rotary bearing mount_v3 (Autodesk Fusion 360 design; units mm, degrees)
Autodesk Fusion 360 part; units mm, degrees
sketch "Sketch1" plane through (0, 0, 0) normal (0, 0, 1) x (1, 0, 0)
  line L0 (-45, 45) -> (45, 45) construction
  line L1 (45, 45) -> (45, -45) construction
  line L2 (45, -45) -> (-45, -45) construction
  line L3 (-45, -45) -> (-45, 45) construction
  line L4 (-45, 45) -> (45, -45) construction
  line L5 (45, 45) -> (-45, -45) construction
  circle A0 centre (-45, 45) radius 2.9
  circle A1 centre (45, 45) radius 2.9
  circle A2 centre (-45, -45) radius 2.9
  circle A3 centre (45, -45) radius 2.9
  line L6 (-60, 45) -> (60, 45) construction
  line L7 (60, 45) -> (60, -45) construction
  line L8 (60, -45) -> (-60, -45) construction
  line L9 (-60, -45) -> (-60, 45) construction
  line L10 (-60, 45) -> (60, -45) construction
  line L11 (60, 45) -> (-60, -45) construction
  circle A4 centre (-60, 45) radius 2.75
  circle A5 centre (60, 45) radius 2.75
  circle A6 centre (60, -45) radius 2.75
  circle A7 centre (-60, -45) radius 2.75
  line L12 (-67.5, 52.5) -> (67.5, 52.5)
  line L13 (67.5, 52.5) -> (67.5, -52.5)
  line L14 (67.5, -52.5) -> (-67.5, -52.5)
  line L15 (-67.5, -52.5) -> (-67.5, 52.5)
  line L16 (-67.5, 52.5) -> (67.5, -52.5) construction
  line L17 (67.5, 52.5) -> (-67.5, -52.5) construction
  circle A8 centre (0, 0) radius 30
  dimension "d1" = 90
  dimension "d2" = 90
  dimension "d3" = 5.8
  dimension "d4" = 5.8
  dimension "d5" = 5.8
  dimension "d6" = 5.8
  dimension "d7" = 120
  dimension "d8" = 90
  dimension "d9" = 5.5
  dimension "d10" = 5.5
  dimension "d11" = 5.5
  dimension "d12" = 5.5
  dimension "d13" = 135
  dimension "d14" = 105
  dimension "d27" = 60
  constraint horizontal L0
  constraint perpendicular L0 L1
  constraint parallel L0 L2
  constraint parallel L1 L3
  constraint coincident L4 A8.centre
  constraint coincident L5 A8.centre
  constraint coincident A8.centre origin
  constraint coincident L0.start L3.end
  constraint coincident L0.end L1.start
  constraint coincident L2.end L3.start
  constraint coincident L1.end L2.start
  constraint horizontal L6
  constraint perpendicular L6 L7
  constraint parallel L6 L8
  constraint parallel L7 L9
  constraint coincident L10 A8.centre
  constraint coincident L11 A8.centre
  constraint coincident L6.start L9.end
  constraint coincident L6.end L7.start
  constraint coincident L7.end L8.start
  constraint coincident L8.end L9.start
  constraint horizontal L12
  constraint perpendicular L12 L13
  constraint parallel L12 L14
  constraint parallel L13 L15
  constraint coincident L16 A8.centre
  constraint coincident L17 A8.centre
  measures "d1" distance of L1.end L2.end
  measures "d2" distance of L0.end L1.end
  measures "d3" diameter of A0
  measures "d4" diameter of A1
  measures "d5" diameter of A2
  measures "d6" diameter of A3
  measures "d7" distance of L7.end L8.end
  measures "d8" distance of L6.end L7.end
  measures "d9" diameter of A4
  measures "d10" diameter of A5
  measures "d11" diameter of A6
  measures "d12" diameter of A7
  measures "d13" distance of L13.end L14.end
  measures "d14" distance of L12.end L13.end
  measures "d27" diameter of A8
extrude "Extrude1" add sketch "Sketch1" along normal blind 3.6
sketch "Sketch2" plane through (0, 0, 0) normal (0, 0, -1) x (1, 0, 0)
  circle A0 centre (-45, -45) radius 2.9
  circle A1 centre (-60, -45) radius 2.75
  circle A2 centre (60, -45) radius 2.75
  circle A3 centre (-60, 45) radius 2.75
  circle A4 centre (45, -45) radius 2.9
  circle A5 centre (-45, 45) radius 2.9
  circle A6 centre (45, 45) radius 2.9
  circle A7 centre (60, 45) radius 2.75
  line L0 (67.5, 52.5) -> (-67.5, 52.5)
  line L1 (-67.5, 52.5) -> (-67.5, -52.5)
  line L2 (-67.5, -52.5) -> (67.5, -52.5)
  line L3 (67.5, -52.5) -> (67.5, 52.5)
  line L4 (-67.5, 52.5) -> (67.5, 52.5)
  line L5 (67.5, 52.5) -> (67.5, -52.5)
  line L6 (67.5, -52.5) -> (-67.5, -52.5)
  line L7 (-67.5, -52.5) -> (-67.5, 52.5)
  line L8 (-67.5, 52.5) -> (67.5, -52.5) construction
  line L9 (67.5, 52.5) -> (-67.5, -52.5) construction
  circle A8 centre (0, 0) radius 30
  dimension "d17" = 135
  dimension "d18" = 105
  constraint horizontal L4
  constraint perpendicular L4 L5
  constraint parallel L4 L6
  constraint parallel L5 L7
  constraint coincident L8 A8.centre
  constraint coincident L9 A8.centre
  constraint coincident A8.centre origin
  measures "d17" distance of L2.end L1.end
  measures "d18" distance of L0.start L2.end
extrude "Extrude2" add sketch "Sketch2" along normal blind 0.2 contours A0 | A4 | A5 | A6 | L0 L1 L2 L3 L4 L5 L6 L7
sketch "Sketch3" plane through (0, 0, -0.2) normal (0, 0, -1) x (1, 0, 0)
  circle A0 centre (-60, -45) radius 2.75
  circle A1 centre (60, -45) radius 2.75
  circle A2 centre (-60, 45) radius 2.75
  circle A3 centre (60, 45) radius 2.75
  line L0 (-67.5, -52.5) -> (67.5, -52.5)
  line L1 (67.5, -52.5) -> (67.5, 52.5)
  line L2 (67.5, 52.5) -> (-67.5, 52.5)
  line L3 (-67.5, 52.5) -> (-67.5, -52.5)
  line L4 (-42.6329, 40.9) -> (-40.2657, 45)
  line L5 (-40.2657, 45) -> (-42.6329, 49.1)
  line L6 (-42.6329, 49.1) -> (-47.3671, 49.1)
  line L7 (-47.3671, 49.1) -> (-49.7343, 45)
  line L8 (-49.7343, 45) -> (-47.3671, 40.9)
  line L9 (-47.3671, 40.9) -> (-42.6329, 40.9)
  line L10 (-47.3671, -40.9) -> (-49.7343, -45)
  line L11 (-49.7343, -45) -> (-47.3671, -49.1)
  line L12 (-47.3671, -49.1) -> (-42.6329, -49.1)
  line L13 (-42.6329, -49.1) -> (-40.2657, -45)
  line L14 (-40.2657, -45) -> (-42.6329, -40.9)
  line L15 (-42.6329, -40.9) -> (-47.3671, -40.9)
  line L16 (47.3671, 40.9) -> (49.7343, 45)
  line L17 (49.7343, 45) -> (47.3671, 49.1)
  line L18 (47.3671, 49.1) -> (42.6329, 49.1)
  line L19 (42.6329, 49.1) -> (40.2657, 45)
  line L20 (40.2657, 45) -> (42.6329, 40.9)
  line L21 (42.6329, 40.9) -> (47.3671, 40.9)
  line L22 (42.6329, -40.9) -> (40.2657, -45)
  line L23 (40.2657, -45) -> (42.6329, -49.1)
  line L24 (42.6329, -49.1) -> (47.3671, -49.1)
  line L25 (47.3671, -49.1) -> (49.7343, -45)
  line L26 (49.7343, -45) -> (47.3671, -40.9)
  line L27 (47.3671, -40.9) -> (42.6329, -40.9)
  circle A4 centre (0, 0) radius 30
  point P0 (-45, 45)
  point P1 (-45, -45)
  point P2 (45, 45)
  point P3 (45, -45)
  dimension "d21" = 4.1
  dimension "d22" = 4.1
  dimension "d23" = 4.1
  dimension "d24" = 4.1
  measures "d21" distance of P0 L9
  measures "d22" distance of P1 L15
  measures "d23" distance of P2 L21
  measures "d24" distance of P3 L27
extrude "Extrude3" add sketch "Sketch3" along normal blind 3.6
sketch "Sketch4" plane through (-67.5, 0, 0) normal (-1, 0, 0) x (0, -1, 0)
  line L0 (52.5, -3.8) -> (52.5, 3.6)
  line L1 (52.5, 3.6) -> (-52.5, 3.6)
  line L2 (-52.5, 3.6) -> (-52.5, -3.8)
  line L3 (-52.5, -3.8) -> (52.5, -3.8)
  line L4 (-3.0507, 8.6121) -> (-4.3315, 9.8929)
  line L5 (-4.8314, 10.1) -> (-3.6911, 10.1) construction
  line L6 (-4.8314, 10.1) -> (-4.5386, 10.1) construction
  line L7 (4.3315, 9.8929) -> (3.0507, 8.6121)
  line L8 (-3.0507, 8.6121) -> (3.0507, 8.6121)
  line L9 (4.8314, 10.1) -> (4.5386, 10.1) construction
  line L10 (4.3315, 9.8929) -> (4.5386, 10.1)
  line L11 (-4.3315, 9.8929) -> (-4.5386, 10.1)
  line L12 (-52.5, -0.1) -> (-45, -0.1) construction
  line L13 (52.5, -0.1) -> (45, -0.1) construction
  constraint coincident L6.end L5
  constraint horizontal L8
  constraint coincident L8.end L7
  constraint midpoint L2 L12.start
  constraint perpendicular L2 L12
  constraint midpoint L0 L13.start
  constraint perpendicular L0 L13
sketch "Sketch5" plane through (0, -52.5, 0) normal (0, -1, 0) x (1, 0, 0)
  line L0 (67.5, -3.8) -> (67.5, 3.6)
  line L1 (67.5, 3.6) -> (-67.5, 3.6)
  line L2 (-67.5, 3.6) -> (-67.5, -3.8)
  line L3 (-67.5, -3.8) -> (67.5, -3.8)
  line L4 (15.1684, -3.7997) -> (16.3088, -3.7997) construction
  line L5 (15.6684, -4.0068) -> (15.4613, -3.7997)
  line L6 (15.1684, -3.7997) -> (15.4613, -3.7997) construction
  line L7 (24.8313, -3.7997) -> (24.5385, -3.7997) construction
  line L8 (16.9492, -5.2876) -> (23.0506, -5.2876)
  line L9 (24.3314, -4.0068) -> (24.5385, -3.7997)
  line L10 (24.3314, -4.0068) -> (23.0506, -5.2876)
  line L11 (16.9492, -5.2876) -> (15.6684, -4.0068)
  line L12 (-67.5, -0.1) -> (-60, -0.1) construction
  line L13 (-60, -0.1) -> (60, -0.1) construction
  line L14 (60, -0.1) -> (67.5, -0.1) construction
  line L15 (-60, -0.1) -> (-20, -0.1) construction
  line L16 (60, -0.1) -> (20, -0.1) construction
  line L17 (-20, -0.1) -> (-20, 10.5) construction
  line L18 (16.9492, -5.2876) -> (19.9999, -5.2876) construction
  line L19 (-23.0508, -5.2876) -> (-20.0001, -5.2876) construction
  line L20 (-15.6686, -4.0068) -> (-15.4615, -3.7997)
  line L21 (-24.8316, -3.7997) -> (-23.6912, -3.7997) construction
  line L22 (-23.0508, -5.2876) -> (-16.9494, -5.2876)
  line L23 (-15.6686, -4.0068) -> (-16.9494, -5.2876)
  line L24 (-23.0508, -5.2876) -> (-24.3316, -4.0068)
  line L25 (-24.8316, -3.7997) -> (-24.5387, -3.7997) construction
  line L26 (-24.3316, -4.0068) -> (-24.5387, -3.7997)
  line L27 (-15.1687, -3.7997) -> (-15.4615, -3.7997) construction
  line L28 (64.8313, -3.7997) -> (64.5385, -3.7997) construction
  line L29 (56.9492, -5.2876) -> (59.9999, -5.2876) construction
  line L30 (64.3314, -4.0068) -> (63.0506, -5.2876)
  line L31 (55.6684, -4.0068) -> (55.4613, -3.7997)
  line L32 (56.9492, -5.2876) -> (55.6684, -4.0068)
  line L33 (55.1684, -3.7997) -> (55.4613, -3.7997) construction
  line L34 (56.9492, -5.2876) -> (63.0506, -5.2876)
  line L35 (64.3314, -4.0068) -> (64.5385, -3.7997)
  line L36 (55.1684, -3.7997) -> (56.3088, -3.7997) construction
  line L37 (-63.0508, -5.2876) -> (-64.3316, -4.0068)
  line L38 (-63.0508, -5.2876) -> (-60.0001, -5.2876) construction
  line L39 (-64.3316, -4.0068) -> (-64.5387, -3.7997)
  line L40 (-55.6686, -4.0068) -> (-56.9494, -5.2876)
  line L41 (-63.0508, -5.2876) -> (-56.9494, -5.2876)
  line L42 (-55.6686, -4.0068) -> (-55.4615, -3.7997)
  line L43 (-64.8316, -3.7997) -> (-64.5387, -3.7997) construction
  line L44 (-55.1687, -3.7997) -> (-55.4615, -3.7997) construction
  line L45 (-64.8316, -3.7997) -> (-63.6912, -3.7997) construction
  constraint coincident L5.end L4
  constraint coincident L8.end L10
  constraint midpoint L2 L12.start
  constraint perpendicular L2 L12
  constraint perpendicular L2 L13
  constraint midpoint L0 L14.end
  constraint perpendicular L0 L14
  constraint coincident L13 L15.end
  constraint coincident L13 L16.end
  constraint perpendicular L1 L17
  constraint midpoint L8 L18.end
  constraint coincident L25.end L21
  constraint coincident L22.end L23
  constraint midpoint L19.end L22
  constraint coincident L31.end L36
  constraint coincident L34.end L30
  constraint midpoint L29.end L34
  constraint coincident L39.end L45
  constraint coincident L41.end L40
  constraint midpoint L38.end L41
extrude "Extrude4" add sketch "Sketch5" against normal blind 105 contours L3 L30 L31 L32 L34 L35 | L3 L5 L8 L9 L10 L11 | L3 L37 L39 L40 L41 L42 | L3 L20 L22 L23 L24 L26
extrude "Extrude5" cut sketch "Sketch3" along normal blind 6 contours A0 | A1 | A2 | A3 | A4
